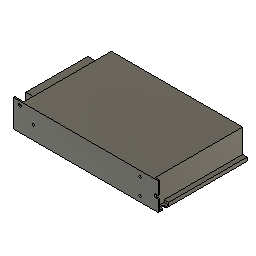
POS-150-C power supply (Autodesk Fusion 360 design; units mm, degrees)
Autodesk Fusion 360 part; units mm, degrees
sketch "Sketch1" plane through (0, 0, 0) normal (0, 0, 1) x (1, 0, 0)
  line L0 (-79.5, 48.75) -> (79.5, 48.75)
  line L1 (79.5, 48.75) -> (79.5, -48.75)
  line L2 (79.5, -48.75) -> (-79.5, -48.75)
  line L3 (-79.5, -48.75) -> (-79.5, 48.75)
  line L4 (-79.5, 0) -> (79.5, 0)
  dimension "d1" = 159
  dimension "d2" = 97.5
  constraint horizontal L0
  constraint vertical L1
  constraint horizontal L2
  constraint vertical L3
  constraint coincident L3 L4.start
  constraint coincident L1 L4.end
  constraint perpendicular L1 L4
  constraint midpoint origin L4
  constraint midpoint L3 L4.start
  measures "d1" distance of L1 L3
  measures "d2" distance of L0 L2
extrude "Extrude1" add sketch "Sketch1" along normal blind 30
sketch "Sketch2" plane through (-79.5, 0, 0) normal (-1, 0, 0) x (0, -1, 0)
  line L0 (-48.75, 0) -> (48.75, 0)
  line L1 (48.75, 0) -> (48.75, 30)
  line L2 (48.75, 30) -> (-48.75, 30)
  line L3 (-48.75, 30) -> (-48.75, 0)
  line L4 (-38, 23) -> (30, 23)
  line L5 (30, 23) -> (30, 6.5)
  line L6 (30, 6.5) -> (-38, 6.5)
  line L7 (-38, 6.5) -> (-38, 23)
  line L8 (-48.75, 30) -> (47.25, 30)
  line L9 (47.25, 30) -> (47.25, 1.5)
  line L10 (47.25, 1.5) -> (-48.75, 1.5)
  line L11 (-48.75, 1.5) -> (-48.75, 30)
  dimension "d5" = 68
  dimension "d6" = 16.5
  dimension "d7" = 10.75
  dimension "d8" = 6.5
  dimension "d9" = 1.5
  dimension "d10" = 1.5
  constraint horizontal L4
  constraint vertical L5
  constraint horizontal L6
  constraint vertical L7
  constraint horizontal L8
  constraint vertical L9
  constraint horizontal L10
  constraint vertical L11
  constraint coincident L2.end L3.start
  measures "d5" distance of L5 L7
  measures "d6" distance of L4 L6
  measures "d7" distance of L3 L7
  measures "d8" distance of L0 L6
  measures "d9" distance of L1 L9
  measures "d10" distance of L0 L10
extrude "Extrude2" cut sketch "Sketch2" against normal blind 10 contours L2 L3 L8 L9 L10 L11
extrude "Extrude3" add 1 faces at (-79.5, 15.3333, 17.5) along direction (-1, 0, 0) blind 5
sketch "Sketch3" plane through (79.5, 0, 0) normal (1, 0, 0) x (0, 1, 0)
  line L0 (-48.75, 0) -> (48.75, 0)
  line L1 (48.75, 0) -> (48.75, 30)
  line L2 (48.75, 30) -> (-48.75, 30)
  line L3 (-48.75, 30) -> (-48.75, 0)
  line L4 (-47.25, 30) -> (48.75, 30)
  line L5 (48.75, 30) -> (48.75, 4)
  line L6 (48.75, 4) -> (-47.25, 4)
  line L7 (-47.25, 4) -> (-47.25, 30)
  dimension "d15" = 1.5
  dimension "d16" = 4
  constraint horizontal L4
  constraint vertical L5
  constraint horizontal L6
  constraint vertical L7
  constraint coincident L1 L5.end
  constraint coincident L2 L4.start
  measures "d15" distance of L3 L7
  measures "d16" distance of L0 L6
extrude "Extrude4" cut sketch "Sketch3" against normal blind 5 contours L1 L2 L4 L5 L6 L7
sketch "Sketch4" plane through (0, 0, 4) normal (0, 0, 1) x (-1, 0, 0)
  line L0 (-79.5, 47.25) -> (-79.5, -48.75)
  line L1 (-79.5, -48.75) -> (-74.5, -48.75)
  line L2 (-74.5, -48.75) -> (-74.5, 47.25)
  line L3 (-74.5, 47.25) -> (-79.5, 47.25)
  line L4 (-79.5, 37.25) -> (-74.5, 37.25)
  dimension "d19" = 10
  constraint coincident L0 L4.start
  constraint coincident L2 L4.end
  constraint perpendicular L2 L4
  measures "d19" distance of L3 L4
extrude "Extrude5" cut sketch "Sketch4" against normal blind 2.5 contours L0 L2 L3 L4
sketch "Sketch5" plane through (0, -48.75, 0) normal (0, -1, 0) x (1, 0, 0)
  line L0 (-79.5, 0) -> (79.5, 0)
  line L1 (79.5, 0) -> (79.5, 30)
  line L2 (79.5, 30) -> (-79.5, 30)
  line L3 (-79.5, 30) -> (-79.5, 0)
  circle A0 centre (-72.5, 26) radius 1.75
  circle A1 centre (76.9, 14.5) radius 1.75
  circle A2 centre (59.5, 23.9) radius 1.25
  circle A3 centre (59.5, 5.9) radius 1.25
  circle A4 centre (-57.5, 15) radius 1.25
  line L4 (76.9, 16.25) -> (79.5, 16.25)
  line L5 (76.9, 12.75) -> (79.5, 12.75)
  dimension "d22" = 2.5
  dimension "d23" = 2.5
  dimension "d24" = 3.5
  dimension "d25" = 2.6
  dimension "d26" = 14.5
  dimension "d27" = 18
  dimension "d28" = 20
  dimension "d29" = 5.9
  dimension "d30" = 20
  dimension "d31" = 137
  dimension "d32" = 15
  dimension "d33" = 3.5
  dimension "d34" = 26
  dimension "d35" = 152
  dimension "d36" = 2.5
  constraint coincident A1 L4.start
  constraint coincident L1 L4.end
  constraint perpendicular L1 L4
  constraint coincident A1 L5.start
  constraint coincident L1 L5.end
  constraint perpendicular L1 L5
  constraint tangent A1 L5
  constraint tangent A1 L4
  measures "d22" diameter of A2
  measures "d23" diameter of A3
  measures "d24" diameter of A1
  measures "d25" distance of L1 A1.centre
  measures "d26" distance of L0 A1.centre
  measures "d27" distance of A2.centre A3.centre
  measures "d28" distance of L1 A3.centre
  measures "d29" distance of L0 A3.centre
  measures "d30" distance of L1 A2.centre
  measures "d31" distance of L1 A4.centre
  measures "d32" distance of L0 A4.centre
  measures "d33" diameter of A0
  measures "d34" distance of L0 A0.centre
  measures "d35" distance of L1 A0.centre
  measures "d36" diameter of A4
extrude "Extrude6" cut sketch "Sketch5" against normal blind 13 contours A0
extrude "Extrude7" cut sketch "Sketch5" against normal blind 5 contours A4
extrude "Extrude8" cut sketch "Sketch5" against normal blind 1.5 contours L1 A1 L4 L5 | A1
extrude "Extrude9" cut sketch "Sketch5" against normal blind 5 contours A3
extrude "Extrude10" cut sketch "Sketch5" against normal blind 5 contours A2
sketch "Sketch6" plane through (0, 0, 0) normal (0, 0, -1) x (1, 0, 0)
  line L0 (79.5, 48.75) -> (-79.5, 48.75)
  line L1 (-79.5, 48.75) -> (-79.5, -48.75)
  line L2 (-79.5, -48.75) -> (79.5, -48.75)
  line L3 (79.5, -48.75) -> (79.5, 48.75)
  circle A0 centre (-75.5, -43.25) radius 1.75
  circle A1 centre (77.75, 42.05) radius 1.75
  line L4 (77.75, 43.8) -> (79.5, 43.8)
  line L5 (77.75, 40.3) -> (79.5, 40.3)
  dimension "d47" = 3.5
  dimension "d48" = 6.7
  dimension "d49" = 1.75
  dimension "d50" = 3.5
  dimension "d51" = 85.3
  dimension "d52" = 155
  constraint coincident A1 L4.start
  constraint coincident L3 L4.end
  constraint perpendicular L3 L4
  constraint coincident A1 L5.start
  constraint coincident L3 L5.end
  constraint perpendicular L3 L5
  constraint tangent A1 L4
  constraint tangent A1 L5
  measures "d47" diameter of A1
  measures "d48" distance of L0 A1.centre
  measures "d49" distance of L3 A1.centre
  measures "d50" diameter of A0
  measures "d51" vertical distance of A0.centre A1.centre
  measures "d52" distance of L3 A0.centre
extrude "Extrude11" cut sketch "Sketch6" against normal blind 7 contours L3 A1 L4 | A1 | L3 A1 L5
extrude "Extrude12" cut sketch "Sketch6" against normal blind 1.5 contours A0
